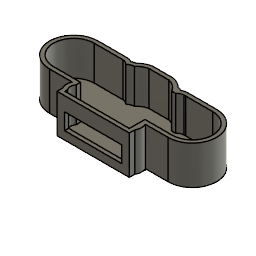
carcasa_camara (Autodesk Fusion 360 archive; units mm, degrees)
design "Ensamble camara 2" references "Raspberry_Pi_Camera_OV5647_IR-CUT_175"
part number: 2026-03-01-18-00-26-014
part number: 2026-03-01-19-10-51-814
Autodesk Fusion 360 part; units mm, degrees
sketch "Boceto1" plane through (0, 0, 0) normal (0, 1, 0) x (1, 0, 0)
  line L0 (16, -17.9) -> (16, -9.75)
  line L1 (30, -10) -> (16.3, -10)
  line L2 (16.3, -10) -> (15.4479, -10)
  arc A0 (30, -10) -> (30, 10) centre (30, 0) ccw
  line L3 (30, 10) -> (16.3, 10)
  line L4 (16.3, 10) -> (15.4479, 10)
  arc A1 (15.4479, 10) -> (13.3557, 4.5) centre (15.4479, 6.8521) ccw
  arc A2 (11.25, 5.0739) -> (5, 12.75) centre (3.4112, 5.0739) ccw
  line L5 (5, 12.75) -> (-5, 12.75)
  arc A3 (-5, 12.75) -> (-11.25, 5.0739) centre (-3.4112, 5.0739) ccw
  line L6 (30, 10.3) -> (16.3, 10.3)
  arc A4 (30, -10.3) -> (30, 10.3) centre (30, 0) ccw
  line L7 (30, -10.3) -> (16.3, -10.3)
  line L8 (16.3, 10.3) -> (15.4479, 10.3)
  line L9 (5.0304, 13.05) -> (-5.0304, 13.05)
  line L10 (-16.3, 10.3) -> (-15.4479, 10.3)
  line L11 (-30, 10.3) -> (-16.3, 10.3)
  arc A5 (-30, 10.3) -> (-30, -10.3) centre (-30, 0) ccw
  line L12 (-30, -10.3) -> (-16.3, -10.3)
  line L13 (-16.3, -18.2) -> (16.3, -18.2)
  line L14 (-16.3, -18.2) -> (-16.3, -16.8323)
  line L15 (-16.3, -12.4677) -> (-16.3, -10.3)
  arc A6 (-16.3, -12.4677) -> (-16.3, -16.8323) centre (-13.5, -14.65) ccw
  line L16 (16.3, -18.2) -> (16.3, -10.3)
  arc A7 (15.4479, 10.3) -> (12.6741, 8.9) centre (15.4479, 6.8521) ccw
  arc A8 (10.5946, 8.9) -> (5.0304, 13.05) centre (3.4112, 5.0739) ccw
  line L17 (10.5946, 8.9) -> (12.6741, 8.9)
  arc A9 (-5.0304, 13.05) -> (-9.6447, 10.3068) centre (-3.4112, 5.0739) ccw
  line L18 (-12.5, 8.9) -> (-12.4552, 8.9)
  arc A10 (-12.7656, 9.0184) -> (-15.4479, 10.3) centre (-15.4479, 6.8521) ccw
  spline S0 degree 3 poles (-12.7656, 9.0184) (-12.3372, 9.4337) (-11.8229, 9.7593) (-11.2592, 9.973) (-10.7536, 10.1646) (-10.2129, 10.2712) (-9.6447, 10.3068) knots 0.554104 0.554104 0.554104 0.554104 0.75 0.75 0.75 0.925678 0.925678 0.925678 0.925678
  line L19 (30, 12.3) -> (16.3, 12.3)
  arc A11 (30, -12.3) -> (30, 12.3) centre (30, 0) ccw
  line L20 (30, -12.3) -> (18.3, -12.3)
  line L21 (16.3, 12.3) -> (15.4479, 12.3)
  arc A12 (15.4479, 12.3) -> (11.8018, 10.9) centre (15.4479, 6.8521) ccw
  line L22 (11.7089, 10.9) -> (11.8018, 10.9)
  arc A13 (11.7089, 10.9) -> (5.2203, 15.05) centre (3.4112, 5.0739) ccw
  line L23 (5.2203, 15.05) -> (-5.2203, 15.05)
  arc A14 (-5.2203, 15.05) -> (-10.6173, 12.2061) centre (-3.4112, 5.0739) ccw
  spline S1 degree 3 poles (-12.6606, 11.533) (-12.4365, 11.6496) (-12.2053, 11.7532) (-11.9681, 11.8431) (-11.5252, 12.011) (-11.0722, 12.1294) (-10.6173, 12.2061) knots 0.693075 0.693075 0.693075 0.693075 0.75 0.75 0.75 0.858412 0.858412 0.858412 0.858412
  arc A15 (-12.6606, 11.533) -> (-15.4479, 12.3) centre (-15.4479, 6.8521) ccw
  line L24 (-16.3, 12.3) -> (-15.4479, 12.3)
  line L25 (-30, 12.3) -> (-16.3, 12.3)
  arc A16 (-30, 12.3) -> (-30, -12.3) centre (-30, 0) ccw
  line L26 (-30, -12.3) -> (-18.5279, -12.3)
  arc A17 (-18.5279, -12.3) -> (-18.3, -17.4361) centre (-13.5, -14.65) ccw
  line L27 (-18.3, -20.2) -> (-18.3, -17.4361)
  line L28 (-18.3, -20.2) -> (18.3, -20.2)
  line L29 (18.3, -20.2) -> (18.3, -12.3)
  dimension "d1" = -0.3
  dimension "d12" = 2
  dimension "d13" = 2
  constraint collinear L14 L15
  constraint tangent L8 A7
  constraint concentric A2 A8
  constraint concentric A3 A9
  constraint tangent L10 A10
  constraint tangent L11 A5
  constraint tangent A5 L12
  constraint concentric A6 A17
  constraint concentric A4 A11
sketch "Boceto2" plane through (0, 0, 0) normal (1, 0, 0) x (0, 0, -1)
  line L0 (0, 25) -> (6.2481, 25) construction
  line L1 (12.3, 0) -> (-12.3, 0)
  line L2 (7.5, -4) -> (3, -4) construction
  point P0 (5.0739, 0)
  dimension "d17" = 25
  dimension "d18" = 4
  constraint horizontal L0
  constraint horizontal L2
  measures "d17" distance of L0 L1
  measures "d18" distance of L2 P0
extrude "Extruir1" add sketch "Boceto1" along normal blind 13.5 and the other way blind 0 makes body 1
extrude "Extruir2" add sketch "Boceto1" against normal blind 4 bodies 1
sketch "Boceto3" plane through (0, -4, 0) normal (0, -1, 0) x (1, 0, 0)
  arc A0 (30, -12.3) -> (30, 12.3) centre (30, 0) ccw
  line L0 (30, 12.3) -> (18.3, 12.3)
  line L1 (18.3, 20.2) -> (18.3, 12.3)
  line L2 (-18.3, 20.2) -> (18.3, 20.2)
  line L3 (-18.3, 20.2) -> (-18.3, 17.4361)
  arc A1 (-18.3, 17.4361) -> (-18.5279, 12.3) centre (-13.5, 14.65) ccw
  line L4 (-30, 12.3) -> (-18.5279, 12.3)
  arc A2 (-30, 12.3) -> (-30, -12.3) centre (-30, 0) ccw
  line L5 (-30, -12.3) -> (-16.3, -12.3)
  line L6 (-16.3, -12.3) -> (-15.4479, -12.3)
  arc A3 (-15.4479, -12.3) -> (-12.6606, -11.533) centre (-15.4479, -6.8521) ccw
  spline S0 degree 3 poles (-12.6606, -11.533) (-12.4365, -11.6496) (-12.2053, -11.7532) (-11.9681, -11.8431) (-11.5252, -12.011) (-11.0722, -12.1294) (-10.6173, -12.2061) knots 0.693075 0.693075 0.693075 0.693075 0.75 0.75 0.75 0.858412 0.858412 0.858412 0.858412
  arc A4 (-10.6173, -12.2061) -> (-5.2203, -15.05) centre (-3.4112, -5.0739) ccw
  line L7 (5.2203, -15.05) -> (-5.2203, -15.05)
  arc A5 (5.2203, -15.05) -> (11.7089, -10.9) centre (3.4112, -5.0739) ccw
  arc A6 (11.8018, -10.9) -> (15.4479, -12.3) centre (15.4479, -6.8521) ccw
  line L8 (30, -12.3) -> (16.3, -12.3)
  line L9 (16.3, -12.3) -> (15.4479, -12.3)
extrude "Extruir3" add 1 faces at (-5.4333, -4, 19.5333) along direction (0, -1, 0) blind 2 on bodies 1 bodies 1
sketch "Boceto4" plane through (0, -6, 0) normal (0, -1, 0) x (1, 0, 0)
  arc A0 (-30, 10.3) -> (-30, -10.3) centre (-30, 0) ccw
  line L0 (-30, 10.3) -> (-16.3, 10.3)
  line L1 (-16.3, 10.3) -> (-16.3, 12.4677)
  arc A1 (-16.3, 16.8323) -> (-16.3, 12.4677) centre (-13.5, 14.65) ccw
  line L2 (-16.3, 16.8323) -> (-16.3, 18.2)
  line L3 (-16.3, 18.2) -> (16.3, 18.2)
  line L4 (16.3, 18.2) -> (16.3, 10.3)
  line L5 (16.3, 10.3) -> (30, 10.3)
  arc A2 (30, -10.3) -> (30, 10.3) centre (30, 0) ccw
  line L6 (30, -10.3) -> (16.3, -10.3)
  line L7 (16.3, -10.3) -> (15.4479, -10.3)
  arc A3 (12.6741, -8.9) -> (15.4479, -10.3) centre (15.4479, -6.8521) ccw
  line L8 (12.6741, -8.9) -> (10.5946, -8.9)
  arc A4 (5.0304, -13.05) -> (10.5946, -8.9) centre (3.4112, -5.0739) ccw
  line L9 (5.0304, -13.05) -> (-5.0304, -13.05)
  arc A5 (-9.6447, -10.3068) -> (-5.0304, -13.05) centre (-3.4112, -5.0739) ccw
  spline S0 degree 3 poles (-9.6447, -10.3068) (-10.2129, -10.2712) (-10.7536, -10.1646) (-11.2592, -9.973) (-11.8229, -9.7593) (-12.3372, -9.4337) (-12.7656, -9.0184) knots -0.925678 -0.925678 -0.925678 -0.925678 -0.75 -0.75 -0.75 -0.554104 -0.554104 -0.554104 -0.554104
  arc A6 (-15.4479, -10.3) -> (-12.7656, -9.0184) centre (-15.4479, -6.8521) ccw
  line L10 (-15.4479, -10.3) -> (-30, -10.3)
  line L11 (18.3, 20.2) -> (-18.3, 20.2)
  line L12 (-18.3, 20.2) -> (-18.3, 17.4361)
  arc A7 (-18.3, 17.4361) -> (-18.5279, 12.3) centre (-13.5, 14.65) ccw
  line L13 (-18.5279, 12.3) -> (-30, 12.3)
  arc A8 (-30, 12.3) -> (-30, -12.3) centre (-30, 0) ccw
  line L14 (-30, -12.3) -> (-15.4479, -12.3)
  arc A9 (-15.4479, -12.3) -> (-12.6606, -11.533) centre (-15.4479, -6.8521) ccw
  spline S1 degree 3 poles (-12.6606, -11.533) (-12.4365, -11.6496) (-12.2053, -11.7532) (-11.9681, -11.8431) (-11.5252, -12.011) (-11.0722, -12.1294) (-10.6173, -12.2061) knots 0.693075 0.693075 0.693075 0.693075 0.75 0.75 0.75 0.858412 0.858412 0.858412 0.858412
  arc A10 (-10.6173, -12.2061) -> (-5.2203, -15.05) centre (-3.4112, -5.0739) ccw
  line L15 (-5.2203, -15.05) -> (5.2203, -15.05)
  arc A11 (5.2203, -15.05) -> (11.7089, -10.9) centre (3.4112, -5.0739) ccw
  line L16 (11.7089, -10.9) -> (11.8018, -10.9)
  arc A12 (11.8018, -10.9) -> (15.4479, -12.3) centre (15.4479, -6.8521) ccw
  line L17 (15.4479, -12.3) -> (16.3, -12.3)
  line L18 (16.3, -12.3) -> (30, -12.3)
  arc A13 (30, -12.3) -> (30, 12.3) centre (30, 0) ccw
  line L19 (30, 12.3) -> (18.3, 12.3)
  line L20 (18.3, 12.3) -> (18.3, 20.2)
  line L21 (16.3, 18.2) -> (16.3, 10.3)
  line L22 (-16.3, 18.2) -> (16.3, 18.2)
  line L23 (-16.3, 18.2) -> (-16.3, 16.8323)
  arc A14 (-16.3, 16.8323) -> (-16.3, 12.4677) centre (-13.5, 14.65) ccw
  line L24 (-16.3, 12.4677) -> (-16.3, 10.3)
  line L25 (-30, 10.3) -> (-16.3, 10.3)
  arc A15 (-30, 10.3) -> (-30, -10.3) centre (-30, 0) ccw
  line L26 (-30, -10.3) -> (-16.3, -10.3)
  line L27 (-16.3, -10.3) -> (-15.4479, -10.3)
  arc A16 (-15.4479, -10.3) -> (-12.7656, -9.0184) centre (-15.4479, -6.8521) ccw
  spline S2 degree 3 poles (-12.7656, -9.0184) (-12.3372, -9.4337) (-11.8229, -9.7593) (-11.2592, -9.973) (-10.7536, -10.1646) (-10.2129, -10.2712) (-9.6447, -10.3068) knots 0.554104 0.554104 0.554104 0.554104 0.75 0.75 0.75 0.925678 0.925678 0.925678 0.925678
  arc A17 (-9.6447, -10.3068) -> (-5.0304, -13.05) centre (-3.4112, -5.0739) ccw
  line L28 (5.0304, -13.05) -> (-5.0304, -13.05)
  arc A18 (5.0304, -13.05) -> (10.5946, -8.9) centre (3.4112, -5.0739) ccw
  line L29 (10.5946, -8.9) -> (12.6741, -8.9)
  arc A19 (12.6741, -8.9) -> (15.4479, -10.3) centre (15.4479, -6.8521) ccw
  line L30 (16.3, -10.3) -> (15.4479, -10.3)
  line L31 (30, -10.3) -> (16.3, -10.3)
  arc A20 (30, -10.3) -> (30, 10.3) centre (30, 0) ccw
  line L32 (30, 10.3) -> (16.3, 10.3)
extrude "Extruir4" add sketch "Boceto4" against normal blind 2 contours A0 L0 L1 A1 L2 L3 L4 L5 A2 L6 L7 A3 L8 A4 L9 A5 S0 A6 L10 L21 L22 L23 A14 L24 L25 A15 L26 L27 A16 S2 A17 L28 A18 L29 A19 L30 L31 A20 L32 bodies 1
sketch "Boceto5" plane through (0, 0, 20.2) normal (0, 0, 1) x (1, 0, 0)
  line L0 (18.3, -6) -> (18.3, 13.5)
  line L1 (18.3, 13.5) -> (-18.3, 13.5)
  line L2 (-18.3, 13.5) -> (-18.3, -6)
  line L3 (-18.3, -6) -> (18.3, -6)
  line L4 (-14.46, 6.42) -> (14.46, 6.42)
  line L5 (14.46, -6.42) -> (-14.46, -6.42)
  line L6 (-14.46, 6.42) -> (14.46, -6.42) construction
  line L7 (14.46, 6.42) -> (-14.46, -6.42) construction
  line L8 (-11.46, 3.42) -> (11.46, 3.42)
  line L9 (-11.46, 3.42) -> (-11.46, 1.18)
  line L10 (11.46, 1.18) -> (11.46, 3.42)
  line L11 (-14.46, -1.82) -> (14.46, -1.82)
  line L12 (-14.46, -6.42) -> (-14.46, -6)
  line L13 (-14.46, -1.82) -> (-14.46, 6.42)
  line L14 (14.46, 6.42) -> (14.46, -1.82)
  line L15 (14.46, -6) -> (14.46, -6.42)
  dimension "d29" = 3
  dimension "d30" = 3
  dimension "d31" = 3
  dimension "d32" = 3
  constraint horizontal L4
  constraint perpendicular L4 L14
  constraint parallel L4 L5
  constraint parallel L13 L14
  constraint coincident L6 origin
  constraint coincident L7 origin
  constraint perpendicular L11 L14
  constraint coincident L3 L12.end
  constraint collinear L12 L13
  constraint coincident L3 L15.start
  constraint collinear L14 L15
  measures "d29" distance of L4 L8
  measures "d30" distance of L9 L13
  measures "d31" distance of L10 L14
  measures "d32" distance of L9.end L11
extrude "Extruir5" cut sketch "Boceto5" against normal up to surface (2 mm away) contours L4 L11 L13 L14 bodies 1
sketch "Boceto6" plane through (0, 0, 0) normal (1, 0, 0) x (0, 0, -1)
ref_plane "PlanoDeObra1" through (3.1, 0, 0) normal (1, 0, 0) x (0, 1, 0)
sketch "Boceto7" plane through (3.1, 0, 0) normal (1, 0, 0) x (0, 0, -1)
  line L0 (6, -6) -> (-6, -6)
  line L1 (-6, -6) -> (-6, -13)
  line L2 (-1, -18) -> (1, -18)
  line L3 (6, -13) -> (6, -6)
  line L4 (0, -6) -> (0, -16) construction
  arc A0 (1, -18) -> (6, -13) centre (1, -13) ccw
  arc A1 (-6, -13) -> (-1, -18) centre (-1, -13) ccw
  circle A2 centre (0, -13) radius 2.5
  dimension "d36" = 6
  dimension "d37" = 6
  dimension "d38" = 12
  dimension "d39" = 5
  dimension "d40" = 5
  dimension "d41" = 5
  constraint horizontal L0
  constraint vertical L1
  constraint horizontal L2
  constraint vertical L3
  constraint coincident L0 L4.start
  constraint perpendicular L0 L4
  constraint tangent L3 A0
  constraint tangent L2 A0
  constraint tangent L2 A1
  constraint tangent L1 A1
  constraint equal A0 A1
  constraint coincident L4 A2.centre
  measures "d36" distance of L3 L4
  measures "d37" distance of L1 L4
  measures "d38" distance of L0 L2
  measures "d39" radius of A0
  measures "d40" diameter of A2
  measures "d41" distance of L2 A2.centre
extrude "Extruir6" add sketch "Boceto7" along normal blind 4 bodies 1
sketch "Boceto8" plane through (0, 0, 0) normal (1, 0, 0) x (0, 0, -1)
mirror "Simetría1" about plane through (0, 0, 0) normal (1, 0, 0) of bodies 1 merged
fillet "Empalme1" radius 1.5 8 edges at (7.1, -6, 0) (5.1, -6, -6) (3.1, -6, 0) (5.1, -6, 6) (-5.1, -6, 6) (-3.1, -6, 0) (-7.1, -6, 0) (-5.1, -6, -6) on bodies 1
copy_body "Cuerpo - > Comp.1" bodies 1 removing the originals makes body 2 in component "Component"
sketch "Boceto9" plane through (0, 13.5, 0) normal (0, 1, 0) x (-1, 0, 0)
  line L0 (18.3, 17.4361) -> (18.3, 20.2)
  line L1 (18.3, 20.2) -> (-18.3, 20.2)
  line L2 (-18.3, 20.2) -> (-18.3, 17.4361)
  arc A0 (-18.3, 17.4361) -> (-18.5279, 12.3) centre (-13.5, 14.65) ccw
  line L3 (-18.5279, 12.3) -> (-30, 12.3)
  arc A1 (-30, 12.3) -> (-30, -12.3) centre (-30, 0) ccw
  line L4 (-30, -12.3) -> (-16.3, -12.3)
  line L5 (-16.3, -12.3) -> (-15.4479, -12.3)
  arc A2 (-15.4479, -12.3) -> (-12.6606, -11.533) centre (-15.4479, -6.8521) ccw
  spline S0 degree 3 poles (-10.6173, -12.2061) (-11.0722, -12.1294) (-11.5252, -12.011) (-11.9681, -11.8431) (-12.2053, -11.7532) (-12.4365, -11.6496) (-12.6606, -11.533) knots -0.858412 -0.858412 -0.858412 -0.858412 -0.75 -0.75 -0.75 -0.693075 -0.693075 -0.693075 -0.693075
  arc A3 (-10.6173, -12.2061) -> (-5.2203, -15.05) centre (-3.4112, -5.0739) ccw
  line L6 (-5.2203, -15.05) -> (5.2203, -15.05)
  arc A4 (5.2203, -15.05) -> (10.6173, -12.2061) centre (3.4112, -5.0739) ccw
  spline S1 degree 3 poles (10.6173, -12.2061) (11.0722, -12.1294) (11.5252, -12.011) (11.9681, -11.8431) (12.2053, -11.7532) (12.4365, -11.6496) (12.6606, -11.533) knots -0.858412 -0.858412 -0.858412 -0.858412 -0.75 -0.75 -0.75 -0.693075 -0.693075 -0.693075 -0.693075
  arc A5 (12.6606, -11.533) -> (15.4479, -12.3) centre (15.4479, -6.8521) ccw
  line L7 (15.4479, -12.3) -> (16.3, -12.3)
  line L8 (16.3, -12.3) -> (30, -12.3)
  arc A6 (30, -12.3) -> (30, 12.3) centre (30, 0) ccw
  line L9 (30, 12.3) -> (18.5279, 12.3)
  arc A7 (18.5279, 12.3) -> (18.3, 17.4361) centre (13.5, 14.65) ccw
  arc A8 (-10.5946, -8.9) -> (-5.0304, -13.05) centre (-3.4112, -5.0739) ccw
  line L10 (-10.5946, -8.9) -> (-12.6741, -8.9)
  arc A9 (-12.7656, -9.0184) -> (-12.6741, -8.9) centre (-15.4479, -6.8521) ccw
  arc A10 (-15.4479, -10.3) -> (-12.7656, -9.0184) centre (-15.4479, -6.8521) ccw
  line L11 (-15.4479, -10.3) -> (-16.3, -10.3)
  line L12 (-16.3, -10.3) -> (-30, -10.3)
  arc A11 (-30, 10.3) -> (-30, -10.3) centre (-30, 0) ccw
  line L13 (-30, 10.3) -> (-16.3, 10.3)
  line L14 (-16.3, 10.3) -> (-16.3, 12.4677)
  line L15 (-16.3, 12.4677) -> (-16.3, 18.2)
  line L16 (-16.3, 18.2) -> (16.3, 18.2)
  line L17 (16.3, 18.2) -> (16.3, 16.8323)
  line L18 (16.3, 16.8323) -> (16.3, 12.4677)
  line L19 (16.3, 12.4677) -> (16.3, 10.3)
  line L20 (16.3, 10.3) -> (30, 10.3)
  arc A12 (30, -10.3) -> (30, 10.3) centre (30, 0) ccw
  line L21 (30, -10.3) -> (16.3, -10.3)
  line L22 (16.3, -10.3) -> (15.4479, -10.3)
  arc A13 (12.7656, -9.0184) -> (15.4479, -10.3) centre (15.4479, -6.8521) ccw
  arc A14 (12.6741, -8.9) -> (12.7656, -9.0184) centre (15.4479, -6.8521) ccw
  line L23 (12.6741, -8.9) -> (10.5946, -8.9)
  arc A15 (5.0304, -13.05) -> (10.5946, -8.9) centre (3.4112, -5.0739) ccw
  line L24 (5.0304, -13.05) -> (-5.0304, -13.05)
  circle A16 centre (13.5, 14.65) radius 3.25
  line L25 (16.3, 12.4677) -> (16.3, 13)
  line L26 (16.3, 16.3) -> (16.3, 16.8323)
  arc A17 (16.3, 12.4677) -> (16.3, 16.8323) centre (13.5, 14.65) ccw
  constraint coincident L18.end L19.start
  constraint coincident A16 L25.end
  constraint coincident L18 L25.end
  constraint parallel L18 L25
  constraint concentric A16 A17
extrude "Extruir1'" cut sketch "Boceto9" against normal up to surface (17.5 mm away) contours L18 A16 L25 L26 A17 | L18 A16 picked at (16.3647, 14.2288) bodies 2 in component "Component"
sketch "Boceto10" plane through (0, 13.5, 0) normal (0, 1, 0) x (-1, 0, 0)
  arc A0 (16.3, 12.4677) -> (16.3, 16.8323) centre (13.5, 14.65) ccw
  line L0 (16.3, 12.4677) -> (16.3, 10.3)
  line L1 (16.3, 10.3) -> (30, 10.3)
  arc A1 (30, -10.3) -> (30, 10.3) centre (30, 0) ccw
  line L2 (30, -10.3) -> (16.3, -10.3)
  line L3 (16.3, -10.3) -> (15.4479, -10.3)
  arc A2 (12.7656, -9.0184) -> (15.4479, -10.3) centre (15.4479, -6.8521) ccw
  arc A3 (12.6741, -8.9) -> (12.7656, -9.0184) centre (15.4479, -6.8521) ccw
  line L4 (12.6741, -8.9) -> (10.5946, -8.9)
  arc A4 (5.0304, -13.05) -> (10.5946, -8.9) centre (3.4112, -5.0739) ccw
  line L5 (5.0304, -13.05) -> (-5.0304, -13.05)
  arc A5 (-10.5946, -8.9) -> (-5.0304, -13.05) centre (-3.4112, -5.0739) ccw
  line L6 (-10.5946, -8.9) -> (-12.6741, -8.9)
  arc A6 (-12.7656, -9.0184) -> (-12.6741, -8.9) centre (-15.4479, -6.8521) ccw
  arc A7 (-15.4479, -10.3) -> (-12.7656, -9.0184) centre (-15.4479, -6.8521) ccw
  line L7 (-15.4479, -10.3) -> (-16.3, -10.3)
  line L8 (-16.3, -10.3) -> (-30, -10.3)
  arc A8 (-30, 10.3) -> (-30, -10.3) centre (-30, 0) ccw
  line L9 (-30, 10.3) -> (-16.3, 10.3)
  line L10 (-16.3, 10.3) -> (-16.3, 12.4677)
  line L11 (-16.3, 12.4677) -> (-16.3, 18.2)
  line L12 (-16.3, 18.2) -> (16.3, 18.2)
  line L13 (16.3, 18.2) -> (16.3, 16.8323)
  line L14 (18.3, 17.4361) -> (18.3, 20.2)
  line L15 (18.3, 20.2) -> (-18.3, 20.2)
  line L16 (-18.3, 20.2) -> (-18.3, 17.4361)
  arc A9 (-18.3, 17.4361) -> (-18.5279, 12.3) centre (-13.5, 14.65) ccw
  line L17 (-18.5279, 12.3) -> (-30, 12.3)
  arc A10 (-30, 12.3) -> (-30, -12.3) centre (-30, 0) ccw
  line L18 (-30, -12.3) -> (-16.3, -12.3)
  line L19 (-16.3, -12.3) -> (-15.4479, -12.3)
  arc A11 (-15.4479, -12.3) -> (-12.6606, -11.533) centre (-15.4479, -6.8521) ccw
  spline S0 degree 3 poles (-10.6173, -12.2061) (-11.0722, -12.1294) (-11.5252, -12.011) (-11.9681, -11.8431) (-12.2053, -11.7532) (-12.4365, -11.6496) (-12.6606, -11.533) knots -0.858412 -0.858412 -0.858412 -0.858412 -0.75 -0.75 -0.75 -0.693075 -0.693075 -0.693075 -0.693075
  arc A12 (-10.6173, -12.2061) -> (-5.2203, -15.05) centre (-3.4112, -5.0739) ccw
  line L20 (-5.2203, -15.05) -> (5.2203, -15.05)
  arc A13 (5.2203, -15.05) -> (10.6173, -12.2061) centre (3.4112, -5.0739) ccw
  spline S1 degree 3 poles (10.6173, -12.2061) (11.0722, -12.1294) (11.5252, -12.011) (11.9681, -11.8431) (12.2053, -11.7532) (12.4365, -11.6496) (12.6606, -11.533) knots -0.858412 -0.858412 -0.858412 -0.858412 -0.75 -0.75 -0.75 -0.693075 -0.693075 -0.693075 -0.693075
  arc A14 (12.6606, -11.533) -> (15.4479, -12.3) centre (15.4479, -6.8521) ccw
  line L21 (15.4479, -12.3) -> (16.3, -12.3)
  line L22 (16.3, -12.3) -> (30, -12.3)
  arc A15 (30, -12.3) -> (30, 12.3) centre (30, 0) ccw
  line L23 (30, 12.3) -> (18.5279, 12.3)
  arc A16 (18.5279, 12.3) -> (18.3, 17.4361) centre (13.5, 14.65) ccw
  line L24 (12.6741, -8.9) -> (10.5946, -8.9)
  arc A17 (5.0304, -13.05) -> (10.5946, -8.9) centre (3.4112, -5.0739) ccw
  spline S2 degree 3 poles (12.7656, -9.0184) (12.3372, -9.4337) (11.8229, -9.7593) (11.2592, -9.973) (10.7536, -10.1646) (10.2129, -10.2712) (9.6447, -10.3068) knots 0.554104 0.554104 0.554104 0.554104 0.75 0.75 0.75 0.925678 0.925678 0.925678 0.925678
  line L25 (12.6741, -8.9) -> (10.5946, -8.9)
  constraint coincident A4 S2.end
  constraint coincident A3.start L4.start
  constraint coincident L4.end A4.end
extrude "Extruir2'" cut sketch "Boceto10" against normal up to surface (17.5 mm away) contours A3 L4 A4 L24 A17 S2 L25 bodies 2 in component "Component"
component "Component" placed x (1, 0, 0) y (0, 1, 0) z (0, 0, 1) at (0, 0, 0)
